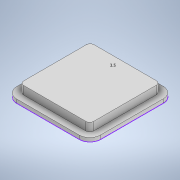
# Autodesk Inventor part: Plug
Saved by Autodesk Inventor 2020 (Build 240168000, 168)
## iProperties
Created: 2021-06-09
Part Number: Plug
Material: Generic
Document SubType Name: Modeling
Designer: Luke
Density: 1 g/cm^3
Appearance: Default
Author: Luke
Autodesk Inventor part; units mm, degrees
ref_plane "YZ Plane" through (0, 0, 0) normal (1, 0, 0) x (0, 1, 0)
ref_plane "XZ Plane" through (0, 0, 0) normal (0, 1, 0) x (-1, 0, 0)
ref_plane "XY Plane" through (0, 0, 0) normal (0, 0, 1) x (1, 0, 0)
sketch "Sketch1" plane through (0, 0, 0) normal (0, 1, 0) x (-1, 0, 0)
  line L0 (63.5, -48.133) -> (79.8363, -48.133)
  line L1 (46.2829, -48.133) -> (63.5, -48.133)
  line L2 (43.9969, -84.201) -> (43.9969, -50.419)
  line L3 (63.5, -86.487) -> (46.2829, -86.487)
  line L4 (79.8363, -86.487) -> (63.5, -86.487)
  line L5 (82.1223, -50.419) -> (82.1223, -84.201)
  arc A0 (79.8363, -86.487) -> (82.1223, -84.201) centre (79.8363, -84.201) ccw
  arc A1 (82.1223, -50.419) -> (79.8363, -48.133) centre (79.8363, -50.419) ccw
  arc A2 (46.2829, -48.133) -> (43.9969, -50.419) centre (46.2829, -50.419) ccw
  arc A3 (43.9969, -84.201) -> (46.2829, -86.487) centre (46.2829, -84.201) ccw
  line L6 (63.5, -89.987) -> (46.2829, -89.987)
  arc A4 (40.4969, -84.201) -> (46.2829, -89.987) centre (46.2829, -84.201) ccw
  line L7 (40.4969, -84.201) -> (40.4969, -50.419)
  arc A5 (46.2829, -44.633) -> (40.4969, -50.419) centre (46.2829, -50.419) ccw
  line L8 (46.2829, -44.633) -> (63.5, -44.633)
  line L9 (63.5, -44.633) -> (79.8363, -44.633)
  arc A6 (85.6223, -50.419) -> (79.8363, -44.633) centre (79.8363, -50.419) ccw
  line L10 (85.6223, -50.419) -> (85.6223, -84.201)
  arc A7 (79.8363, -89.987) -> (85.6223, -84.201) centre (79.8363, -84.201) ccw
  line L11 (79.8363, -89.987) -> (63.5, -89.987)
  dimension "d4" = 3.5
  constraints: 24 end point, 16 point on circle, 8 centre point, 9 other
  measures "d4" distance between parallel lines of L4 L11
extrude "Extrusion1" add sketch "Sketch1" along normal blind 2 contours L0 A1 L5 A0 L4 L3 A3 L2 A2 L1 | L6 A4 L7 A5 L8 L9 A6 L10 A7 L11
sketch "Sketch3" plane through (0, 2, 0) normal (0, 1, 0) x (1, 0, 0)
  line L0 (-82.1223, 50.419) -> (-82.1223, 84.201) projected
  arc A0 (-82.1223, 50.419) -> (-79.8363, 48.133) centre (-79.8363, 50.419) ccw projected
  line L1 (-63.5, 48.133) -> (-79.8363, 48.133) projected
  line L2 (-46.2829, 48.133) -> (-63.5, 48.133) projected
  arc A1 (-46.2829, 48.133) -> (-43.9969, 50.419) centre (-46.2829, 50.419) ccw projected
  line L3 (-43.9969, 84.201) -> (-43.9969, 50.419) projected
  arc A2 (-43.9969, 84.201) -> (-46.2829, 86.487) centre (-46.2829, 84.201) ccw projected
  line L4 (-63.5, 86.487) -> (-46.2829, 86.487) projected
  line L5 (-79.8363, 86.487) -> (-63.5, 86.487) projected
  arc A3 (-79.8363, 86.487) -> (-82.1223, 84.201) centre (-79.8363, 84.201) ccw projected
  line L6 (-63.5, 86.287) -> (-46.2829, 86.287)
  arc A4 (-44.1969, 84.201) -> (-46.2829, 86.287) centre (-46.2829, 84.201) ccw
  line L7 (-44.1969, 84.201) -> (-44.1969, 50.419)
  arc A5 (-46.2829, 48.333) -> (-44.1969, 50.419) centre (-46.2829, 50.419) ccw
  line L8 (-46.2829, 48.333) -> (-63.5, 48.333)
  line L9 (-63.5, 48.333) -> (-79.8363, 48.333)
  arc A6 (-81.9223, 50.419) -> (-79.8363, 48.333) centre (-79.8363, 50.419) ccw
  line L10 (-81.9223, 50.419) -> (-81.9223, 84.201)
  arc A7 (-79.8363, 86.287) -> (-81.9223, 84.201) centre (-79.8363, 84.201) ccw
  line L11 (-79.8363, 86.287) -> (-63.5, 86.287)
  dimension "d7" = 0.2
  constraints: 12 end point, 8 point on circle, 4 centre point, 9 other
  measures "d7" distance between parallel lines of L5 L11
extrude "Extrusion3" add sketch "Sketch3" along normal blind 4.484 contours L6 A4 L7 A5 L8 L9 A6 L10 A7 L11
body "Solid1"
